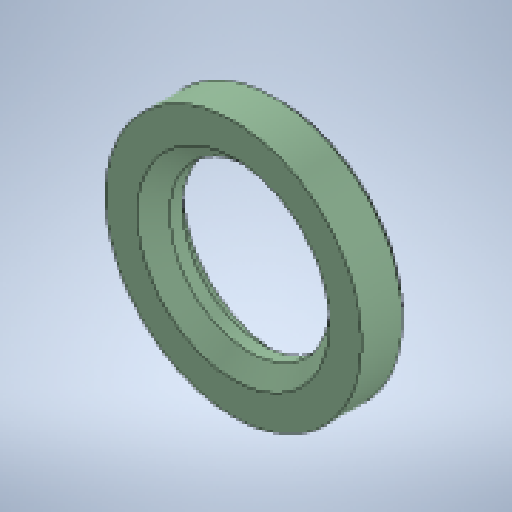
# Autodesk Inventor part: Tire
Saved by Autodesk Inventor 2023.2 (Build 272271000, 271)
## iProperties
Created: 2023-02-06
Part Number: Tire
Material: Rubber, Silicone
Document SubType Name: Modeling
Designer: Nathan Cai
Density: 1.25 g/cm^3
Appearance: Rubber - Green
Mass: 12.3222 g
Surface Area: 43.559 cm^2
Volume: 9.85775 cm^3
Author: Nathan Cai
Autodesk Inventor part; units mm, degrees
ref_plane "YZ Plane" through (0, 0, 0) normal (1, 0, 0) x (0, 1, 0)
ref_plane "XZ Plane" through (0, 0, 0) normal (0, 1, 0) x (-1, 0, 0)
ref_plane "XY Plane" through (0, 0, 0) normal (0, 0, 1) x (1, 0, 0)
sketch "Sketch1" plane through (0, 0, 0) normal (0, 0, 1) x (1, 0, 0)
  circle A0 centre (0, 0) radius 15.875
  circle A1 centre (0, 0) radius 25.4
  dimension "d0" = 31.75
  dimension "d1" = 50.8
  constraints: 2 centre point, 2 coincident
  measures "d0" diameter of A0
  measures "d1" diameter of A1
extrude "Extrusion1" add sketch "Sketch1" along normal blind 8.89
chamfer "Chamfer1" distance 0.7937 angle 45 1 edges at (-25.4, 0, 0)
chamfer "Chamfer2" distance 3.175 angle 45 2 edges at (-15.875, 0, 8.89) (-15.875, 0, 0)
body "Solid1"
